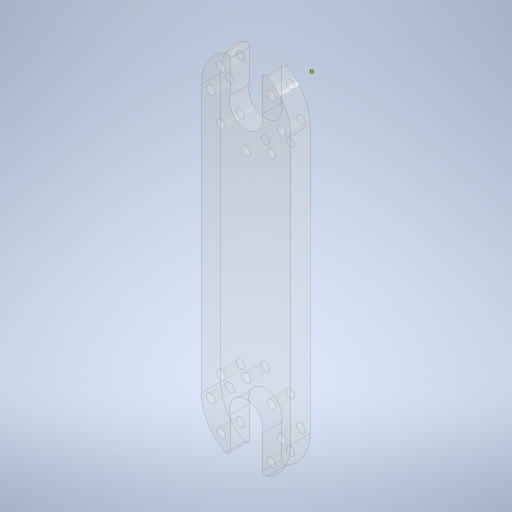
# Autodesk Inventor part: frame_ankle_to_knee1
Saved by Autodesk Inventor 2024 (Build 280153000, 153)
## iProperties
Created: 2024-09-03
Part Number: frame_ankle_to_knee1
Material: PMMA 플라스틱
Document SubType Name: Modeling
Designer: jmha0
Density: 1.188 g/cm^3
Appearance: 폴리카보네이트 - 선명
Mass: 17.1731 g
Surface Area: 75.8237 cm^2
Volume: 14.4555 cm^3
Author: jmha0
Autodesk Inventor part; units mm, degrees
ref_plane "YZ Plane" through (0, 0, 0) normal (1, 0, 0) x (0, 1, 0)
ref_plane "XZ Plane" through (0, 0, 0) normal (0, 1, 0) x (-1, 0, 0)
ref_plane "XY Plane" through (0, 0, 0) normal (0, 0, 1) x (1, 0, 0)
sketch "스케치1" plane through (0, 0, 0) normal (0, 0, 1) x (1, 0, 0)
  circle A0 centre (4.8832, 36.8726) radius 5
  circle A1 centre (4.8832, 47.8726) radius 1.55
  circle A2 centre (4.8832, 36.8726) radius 5
  arc A3 (-0.1168, 38.3009) -> (9.8832, 38.3009) centre (4.8832, 36.8726) ccw
  line L0 (4.8832, 42.0726) -> (9.8832, 42.0726)
  line L1 (4.8832, 42.0726) -> (-0.1168, 42.0726)
  circle A4 centre (4.8832, 36.8726) radius 13.9
  line L2 (9.8832, 42.0726) -> (9.8832, 49.8422)
  line L3 (-0.1168, 42.0726) -> (-0.1168, 49.8422)
  line L4 (9.8832, 42.0726) -> (9.8832, 38.3009)
  line L5 (-0.1168, 42.0726) -> (-0.1168, 38.3009)
  circle A5 centre (4.8832, 36.8726) radius 1.5
  line L6 (18.7832, 36.8726) -> (18.7832, -4.6274)
  line L7 (-9.0168, 36.8726) -> (-9.0168, -4.6274)
  arc A6 (-0.1168, 49.8422) -> (-9.0168, 36.8726) centre (4.8832, 36.8726) ccw
  arc A7 (18.7832, 36.8726) -> (9.8832, 49.8422) centre (4.8832, 36.8726) ccw
  line L8 (-9.0168, -4.6274) -> (18.7832, -4.6274)
  circle A8 centre (4.8832, 36.8726) radius 13.9
  line L9 (-9.0168, -46.1274) -> (-9.0168, -4.6274)
  line L10 (18.7832, -46.1274) -> (18.7832, -4.6274)
  line L11 (18.7832, -4.6274) -> (-9.0168, -4.6274)
  circle A9 centre (-2.895, 44.6508) radius 1.35
  circle A10 centre (-6.1168, 36.8726) radius 1.35
  circle A11 centre (-2.895, 29.0945) radius 1.35
  circle A12 centre (4.8832, 25.8726) radius 1.35
  circle A13 centre (12.6614, 29.0945) radius 1.35
  circle A14 centre (15.8832, 36.8726) radius 1.35
  circle A15 centre (12.6614, 44.6508) radius 1.35
  circle A16 centre (4.8832, -46.1274) radius 5
  circle A17 centre (4.8832, -57.1274) radius 1.55
  circle A18 centre (4.8832, -46.1274) radius 5
  arc A19 (9.8832, -47.5556) -> (-0.1168, -47.5556) centre (4.8832, -46.1274) ccw
  line L12 (4.8832, -51.3274) -> (-0.1168, -51.3274)
  line L13 (4.8832, -51.3274) -> (9.8832, -51.3274)
  line L14 (-0.1168, -51.3274) -> (-0.1168, -59.0969)
  line L15 (9.8832, -51.3274) -> (9.8832, -59.0969)
  line L16 (-0.1168, -51.3274) -> (-0.1168, -47.5556)
  line L17 (9.8832, -51.3274) -> (9.8832, -47.5556)
  circle A20 centre (4.8832, -46.1274) radius 1.5
  circle A21 centre (12.6614, -53.9055) radius 1.35
  circle A22 centre (15.8832, -46.1274) radius 1.35
  circle A23 centre (12.6614, -38.3492) radius 1.35
  circle A24 centre (4.8832, -35.1274) radius 1.35
  circle A25 centre (-2.895, -38.3492) radius 1.35
  circle A26 centre (-6.1168, -46.1274) radius 1.35
  circle A27 centre (-2.895, -53.9055) radius 1.35
  circle A28 centre (4.8832, -46.1274) radius 13.9
  point P0 (0, 0)
  point P1 (18.7832, -4.6274)
  point P2 (18.7832, -46.1274)
  dimension "d0" = 0.2
  dimension "d8" = 41.5
  dimension "d9" = 41.5
  dimension "d13" = 41.5
  dimension "d14" = 41.5
  dimension "d15" = 2.7
  dimension "d16" = 2.7
  dimension "d17" = 2.7
  dimension "d18" = 2.7
  dimension "d19" = 2.7
  dimension "d20" = 2.7
  dimension "d21" = 2.7
  dimension "d24" = 0.2
  dimension "d25" = 2.7
  dimension "d26" = 2.7
  dimension "d27" = 2.7
  dimension "d28" = 2.7
  dimension "d29" = 2.7
  dimension "d30" = 2.7
  dimension "d31" = 2.7
  dimension "d32" = 27.8
  constraints: 36 end point, 28 centre point, 8 point on circle, 7 vertical, 4 coincident, 4 tangent, 1 horizontal, 4 other
  measures "d0" radial gap between concentric circles of A0 A3
  measures "d8" distance of L6.start L6.end
  measures "d9" distance of L7.start L7.end
  measures "d13" distance of L9.start L11.end
  measures "d14" distance of L10.start L10.end
  measures "d15" diameter of A9
  measures "d16" diameter of A10
  measures "d17" diameter of A11
  measures "d18" diameter of A12
  measures "d19" diameter of A13
  measures "d20" diameter of A14
  measures "d21" diameter of A15
  measures "d24" radial gap between concentric circles of A16 A19
  measures "d25" diameter of A21
  measures "d26" diameter of A22
  measures "d27" diameter of A23
  measures "d28" diameter of A24
  measures "d29" diameter of A25
  measures "d30" diameter of A26
  measures "d31" diameter of A27
  measures "d32" diameter of A28
extrude "돌출1" add sketch "스케치1" along normal blind 6 contours A3 L4 L2 A4 L3 L5 | A4 L6 L8 L7 | L8 L10 A28 L9 | A28 L15 L17 A19 L16 L14
fillet "모깎기1" radius 1 4 edges at (-0.1168, 49.8422, 3) (9.8832, 49.8422, 3) (-0.1168, -59.0969, 3) (9.8832, -59.0969, 3)
